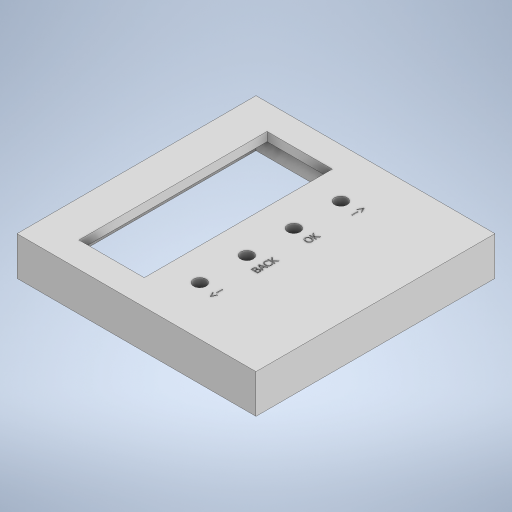
# Autodesk Inventor part: cover pcb
Saved by Autodesk Inventor 2023 (Build 270158030, 158C)
## iProperties
Created: 2023-02-26
Part Number: cover pcb
Material: Generic
Document SubType Name: Modeling
Designer: fatih
Density: 1 g/cm^3
Appearance: Default
Author: fatih
Autodesk Inventor part; units mm, degrees
ref_plane "YZ Plane" through (0, 0, 0) normal (1, 0, 0) x (0, 1, 0)
ref_plane "XZ Plane" through (0, 0, 0) normal (0, 1, 0) x (-1, 0, 0)
ref_plane "XY Plane" through (0, 0, 0) normal (0, 0, 1) x (1, 0, 0)
sketch "Sketch1" plane through (0, 0, 0) normal (0, 1, 0) x (-1, 0, 0)
  line L0 (0, 0) -> (100, 0)
  line L1 (100, 0) -> (100, -100)
  line L2 (100, -100) -> (0, -100)
  line L3 (0, -100) -> (0, 0)
  dimension "d0" = 100
  dimension "d1" = 100
  constraints: 8 end point, 2 parallel, 1 horizontal, 1 perpendicular
  measures "d0" distance of L2.end L0.start
  measures "d1" distance of L0.start L0.end
extrude "Extrusion1" add sketch "Sketch1" along normal blind 13.5
sketch "Sketch2" plane through (0, 13.5, 0) normal (0, 1, 0) x (1, 0, 0)
  line L0 (-100, 100) -> (-100, 0) projected
  line L1 (0, 0) -> (0, 100) projected
  line L2 (-87.5, 50) -> (-87.5, 92.5)
  line L3 (-87.5, 92.5) -> (-87.5, 7.5)
  line L4 (-87.5, 7.5) -> (-58, 7.5)
  line L5 (-58, 7.5) -> (-58, 92.5)
  line L6 (-58, 92.5) -> (-87.5, 92.5)
  dimension "d4" = 42.5
  dimension "d5" = 85
  dimension "d6" = 29.5
  constraints: 10 end point, 3 perpendicular, 1 point on line, 1 vertical
  measures "d4" distance of L2.start L2.end
  measures "d5" distance of L2.end L3.end
  measures "d6" distance of L3.end L4.end
shell "Shell1" thickness 4 outward yes removed faces 1 at (-33.3333, 0, -33.3333)
extrude "Extrusion2" cut sketch "Sketch2" along normal blind 13.5
sketch "Sketch3" plane through (0, 17.5, 0) normal (0, 1, 0) x (1, 0, 0)
  line L0 (-58, 7.5) -> (-58, 92.5) projected
  line L1 (-58, 50) -> (0, 50)
  line L2 (0, 0) -> (0, 100) projected
  line L3 (-29, 50) -> (-58, 50)
  line L4 (-87.5, 7.5) -> (-58, 7.5) projected
  circle A0 centre (-43.5, 81.875) radius 2.85
  circle A1 centre (-43.5, 60.625) radius 2.85
  circle A2 centre (-43.5, 18.125) radius 2.85
  circle A3 centre (-43.5, 39.375) radius 2.85
  dimension "d10" = 5.7
  dimension "d11" = 5.7
  constraints: 4 centre point, 4 end point, 3 midpoint, 2 symmetric about line, 1 collinear, 2 other
  measures "d10" diameter of A0
  measures "d11" diameter of A1
extrude "Extrusion3" cut sketch "Sketch3" against normal blind 13.5
sketch "Sketch5" plane through (0, 17.5, 0) normal (0, 1, 0) x (1, 0, 0)
  circle A0 centre (-43.5, 18.125) radius 2.85 projected
  line L0 (-40.65, 18.125) -> (-40.65, 81.875)
  circle A1 centre (-43.5, 81.875) radius 2.85 projected
  line L1 (-30.65, 18.125) -> (-30.65, 81.875)
  line L2 (-40.65, 81.875) -> (-40.65, 18.125)
  line L3 (-30.65, 15.275) -> (-30.65, 84.725)
  line L4 (-40.65, 84.725) -> (-40.65, 15.275)
  line L5 (-36.861, 14.6566) -> (-36.861, 20.7501) construction
  line L6 (-36.861, 20.7501) -> (-34.517, 20.7501) construction
  line L7 (-34.517, 20.7501) -> (-34.517, 14.6566) construction
  line L8 (-34.517, 14.6566) -> (-36.861, 14.6566) construction
  line L9 (-36.7452, 78.7325) -> (-36.7452, 84.8261) construction
  line L10 (-36.7452, 84.8261) -> (-34.4012, 84.8261) construction
  line L11 (-34.4012, 84.8261) -> (-34.4012, 78.7325) construction
  line L12 (-34.4012, 78.7325) -> (-36.7452, 78.7325) construction
  line L13 (-37.2991, 57.9723) -> (-37.2991, 63.4039) construction
  line L14 (-37.2991, 63.4039) -> (-34.1227, 63.4039) construction
  line L15 (-34.1227, 63.4039) -> (-34.1227, 57.9723) construction
  line L16 (-34.1227, 57.9723) -> (-37.2991, 57.9723) construction
  line L17 (-37.2212, 34.5686) -> (-37.2212, 44.5351) construction
  line L18 (-37.2212, 44.5351) -> (-33.6501, 44.5351) construction
  line L19 (-33.6501, 44.5351) -> (-33.6501, 34.5686) construction
  line L20 (-33.6501, 34.5686) -> (-37.2212, 34.5686) construction
  line L21 (-40.65, 84.725) -> (-40.65, 12.725)
  line L22 (-30.65, 12.725) -> (-30.65, 84.725)
  line L23 (-30.65, 12.725) -> (-30.65, 86.725)
  line L24 (-30.65, 86.725) -> (-40.65, 86.725)
  line L25 (-40.65, 86.725) -> (-40.65, 12.725)
  circle A2 centre (-43.5, 39.375) radius 2.85 projected
  circle A3 centre (-43.5, 60.625) radius 2.85 projected
  line L26 (-34.517, 17.2674) -> (-35.5668, 15.0691)
  line L27 (-35.5668, 15.0691) -> (-35.8113, 15.0691)
  line L28 (-35.8113, 15.0691) -> (-36.861, 17.2674)
  line L29 (-36.861, 17.2674) -> (-36.498, 17.2674)
  line L30 (-36.498, 17.2674) -> (-35.6903, 15.5631)
  line L31 (-35.6903, 15.5631) -> (-34.8801, 17.2674)
  line L32 (-34.8801, 17.2674) -> (-34.517, 17.2674)
  line L33 (-35.505, 19.0458) -> (-35.505, 17.8923)
  line L34 (-35.505, 17.8923) -> (-35.8755, 17.8923)
  line L35 (-35.8755, 17.8923) -> (-35.8755, 19.0458)
  line L36 (-35.8755, 19.0458) -> (-35.505, 19.0458)
  line L37 (-35.505, 20.5673) -> (-35.505, 19.4138)
  line L38 (-35.505, 19.4138) -> (-35.8755, 19.4138)
  line L39 (-35.8755, 19.4138) -> (-35.8755, 20.5673)
  line L40 (-35.8755, 20.5673) -> (-35.505, 20.5673)
  spline S0 degree 2 poles (-35.055, 36.9448) (-34.8278, 36.9448) (-34.4795, 36.7719) (-34.3659, 36.6286) knots 0 0 0 1 2 2 2
  spline S1 degree 2 poles (-34.3659, 36.6286) (-34.2325, 36.4557) (-34.1189, 36.063) (-34.1189, 35.7518) knots 0 0 0 1 2 2 2
  line L41 (-34.1189, 35.7518) -> (-34.1189, 34.8774)
  line L42 (-34.1189, 34.8774) -> (-37.1669, 34.8774)
  line L43 (-37.1669, 34.8774) -> (-37.1669, 35.6851)
  spline S2 degree 2 poles (-37.1669, 35.6851) (-37.1669, 36.0111) (-37.1249, 36.3371) (-37.0434, 36.4853) knots 0 0 0 1 2 2 2
  spline S3 degree 2 poles (-37.0434, 36.4853) (-36.9569, 36.6508) (-36.6729, 36.8015) (-36.4802, 36.8015) knots 0 0 0 1 2 2 2
  spline S4 degree 2 poles (-36.4802, 36.8015) (-36.2653, 36.8015) (-35.9245, 36.5743) (-35.8281, 36.3742) knots 0 0 0 1 2 2 2
  line L44 (-35.8281, 36.3742) -> (-35.8133, 36.3742)
  spline S5 degree 2 poles (-35.8133, 36.3742) (-35.7392, 36.6459) (-35.3465, 36.9448) (-35.055, 36.9448) knots 0 0 0 1 2 2 2
  spline S6 degree 2 poles (-35.0377, 36.5224) (-35.2106, 36.5224) (-35.4329, 36.4236) (-35.512, 36.2754) knots 0 0 0 1 2 2 2
  spline S7 degree 2 poles (-35.512, 36.2754) (-35.5614, 36.1791) (-35.591, 35.9518) (-35.591, 35.7419) knots 0 0 0 1 2 2 2
  line L45 (-35.591, 35.7419) -> (-35.591, 35.2825)
  line L46 (-35.591, 35.2825) -> (-34.4647, 35.2825)
  line L47 (-34.4647, 35.2825) -> (-34.4647, 35.611)
  spline S8 degree 2 poles (-34.4647, 35.611) (-34.4647, 35.8777) (-34.5141, 36.184) (-34.5931, 36.3026) knots 0 0 0 1 2 2 2
  spline S9 degree 2 poles (-34.5931, 36.3026) (-34.6746, 36.4162) (-34.8772, 36.5224) (-35.0377, 36.5224) knots 0 0 0 1 2 2 2
  spline S10 degree 2 poles (-36.4234, 36.3791) (-36.5321, 36.3791) (-36.6951, 36.305) (-36.742, 36.2235) knots 0 0 0 1 2 2 2
  spline S11 degree 2 poles (-36.742, 36.2235) (-36.7964, 36.1247) (-36.8211, 35.8851) (-36.8211, 35.6702) knots 0 0 0 1 2 2 2
  line L48 (-36.8211, 35.6702) -> (-36.8211, 35.2825)
  line L49 (-36.8211, 35.2825) -> (-35.9294, 35.2825)
  line L50 (-35.9294, 35.2825) -> (-35.9294, 35.7419)
  spline S12 degree 2 poles (-35.9294, 35.7419) (-35.9294, 35.9321) (-35.9689, 36.1124) (-36.0307, 36.2087) knots 0 0 0 1 2 2 2
  spline S13 degree 2 poles (-36.0307, 36.2087) (-36.09, 36.3026) (-36.2801, 36.3791) (-36.4234, 36.3791) knots 0 0 0 1 2 2 2
  line L51 (-34.1189, 37.0189) -> (-37.1669, 38.0464)
  line L52 (-37.1669, 38.0464) -> (-37.1669, 38.5453)
  line L53 (-37.1669, 38.5453) -> (-34.1189, 39.5729)
  line L54 (-34.1189, 39.5729) -> (-34.1189, 39.1456)
  line L55 (-34.1189, 39.1456) -> (-34.971, 38.8689)
  line L56 (-34.971, 38.8689) -> (-34.971, 37.7055)
  line L57 (-34.971, 37.7055) -> (-34.1189, 37.4289)
  line L58 (-34.1189, 37.4289) -> (-34.1189, 37.0189)
  line L59 (-35.3168, 38.7578) -> (-36.7519, 38.286)
  line L60 (-36.7519, 38.286) -> (-35.3168, 37.8167)
  line L61 (-35.3168, 37.8167) -> (-35.3168, 38.7578)
  spline S14 degree 2 poles (-34.0645, 41.0524) (-34.0645, 40.756) (-34.2646, 40.2546) (-34.4647, 40.0718) knots 0 0 0 1 2 2 2
  spline S15 degree 2 poles (-34.4647, 40.0718) (-34.6623, 39.889) (-35.2551, 39.689) (-35.6404, 39.689) knots 0 0 0 1 2 2 2
  spline S16 degree 2 poles (-35.6404, 39.689) (-36.0233, 39.689) (-36.5914, 39.8841) (-36.8013, 40.0693) knots 0 0 0 1 2 2 2
  spline S17 degree 2 poles (-36.8013, 40.0693) (-37.0063, 40.2521) (-37.2212, 40.7511) (-37.2212, 41.0598) knots 0 0 0 1 2 2 2
  spline S18 degree 2 poles (-37.2212, 41.0598) (-37.2212, 41.213) (-37.1768, 41.4822) (-37.1422, 41.5958) knots 0 0 0 1 2 2 2
  spline S19 degree 2 poles (-37.1422, 41.5958) (-37.1101, 41.6946) (-37.0187, 41.8996) (-36.9643, 42.0009) knots 0 0 0 1 2 2 2
  line L62 (-36.9643, 42.0009) -> (-36.4753, 42.0009)
  line L63 (-36.4753, 42.0009) -> (-36.4753, 41.9688)
  spline S20 degree 2 poles (-36.4753, 41.9688) (-36.5247, 41.9144) (-36.663, 41.7465) (-36.7297, 41.6255) knots 0 0 0 1 2 2 2
  spline S21 degree 2 poles (-36.7297, 41.6255) (-36.7939, 41.5094) (-36.8754, 41.2352) (-36.8754, 41.0573) knots 0 0 0 1 2 2 2
  spline S22 degree 2 poles (-36.8754, 41.0573) (-36.8754, 40.8622) (-36.7149, 40.5139) (-36.5617, 40.383) knots 0 0 0 1 2 2 2
  spline S23 degree 2 poles (-36.5617, 40.383) (-36.4061, 40.2546) (-35.9343, 40.1113) (-35.6404, 40.1113) knots 0 0 0 1 2 2 2
  spline S24 degree 2 poles (-35.6404, 40.1113) (-35.3267, 40.1113) (-34.8747, 40.262) (-34.7191, 40.3929) knots 0 0 0 1 2 2 2
  spline S25 degree 2 poles (-34.7191, 40.3929) (-34.5684, 40.5214) (-34.4153, 40.8647) (-34.4153, 41.0573) knots 0 0 0 1 2 2 2
  spline S26 degree 2 poles (-34.4153, 41.0573) (-34.4153, 41.2327) (-34.5017, 41.5316) (-34.566, 41.6477) knots 0 0 0 1 2 2 2
  spline S27 degree 2 poles (-34.566, 41.6477) (-34.6302, 41.7588) (-34.7636, 41.9243) (-34.8105, 41.9713) knots 0 0 0 1 2 2 2
  line L64 (-34.8105, 41.9713) -> (-34.8105, 42.0009)
  line L65 (-34.8105, 42.0009) -> (-34.3264, 42.0009)
  spline S28 degree 2 poles (-34.3264, 42.0009) (-34.2794, 41.8996) (-34.193, 41.7218) (-34.1535, 41.5958) knots 0 0 0 1 2 2 2
  spline S29 degree 2 poles (-34.1535, 41.5958) (-34.109, 41.4624) (-34.0645, 41.2352) (-34.0645, 41.0524) knots 0 0 0 1 2 2 2
  line L66 (-34.1189, 44.6018) -> (-34.1189, 44.0757)
  line L67 (-34.1189, 44.0757) -> (-35.5367, 42.9617)
  line L68 (-35.5367, 42.9617) -> (-35.3366, 42.7839)
  line L69 (-35.3366, 42.7839) -> (-34.1189, 42.7839)
  line L70 (-34.1189, 42.7839) -> (-34.1189, 42.3788)
  line L71 (-34.1189, 42.3788) -> (-37.1669, 42.3788)
  line L72 (-37.1669, 42.3788) -> (-37.1669, 42.7839)
  line L73 (-37.1669, 42.7839) -> (-35.7664, 42.7839)
  line L74 (-35.7664, 42.7839) -> (-37.1669, 44.0337)
  line L75 (-37.1669, 44.0337) -> (-37.1669, 44.5277)
  line L76 (-37.1669, 44.5277) -> (-35.8059, 43.2655)
  line L77 (-35.8059, 43.2655) -> (-34.1189, 44.6018)
  spline S30 degree 2 poles (-36.8866, 60.4374) (-36.6841, 60.6103) (-36.0913, 60.8029) (-35.7109, 60.8029) knots 0 0 0 1 2 2 2
  spline S31 degree 2 poles (-35.7109, 60.8029) (-35.3404, 60.8029) (-34.7402, 60.6152) (-34.5377, 60.4374) knots 0 0 0 1 2 2 2
  spline S32 degree 2 poles (-34.5377, 60.4374) (-34.3252, 60.2497) (-34.1227, 59.7532) (-34.1227, 59.4543) knots 0 0 0 1 2 2 2
  spline S33 degree 2 poles (-34.1227, 59.4543) (-34.1227, 59.1456) (-34.3326, 58.6516) (-34.5377, 58.4712) knots 0 0 0 1 2 2 2
  spline S34 degree 2 poles (-34.5377, 58.4712) (-34.7402, 58.2959) (-35.3355, 58.1081) (-35.7109, 58.1081) knots 0 0 0 1 2 2 2
  spline S35 degree 2 poles (-35.7109, 58.1081) (-36.0938, 58.1081) (-36.6767, 58.2983) (-36.8866, 58.4737) knots 0 0 0 1 2 2 2
  spline S36 degree 2 poles (-36.8866, 58.4737) (-37.0892, 58.6516) (-37.2991, 59.148) (-37.2991, 59.4543) knots 0 0 0 1 2 2 2
  spline S37 degree 2 poles (-37.2991, 59.4543) (-37.2991, 59.7655) (-37.0818, 60.2645) (-36.8866, 60.4374) knots 0 0 0 1 2 2 2
  spline S38 degree 2 poles (-35.7109, 60.3806) (-36.0123, 60.3806) (-36.4791, 60.2497) (-36.6322, 60.1311) knots 0 0 0 1 2 2 2
  spline S39 degree 2 poles (-36.6322, 60.1311) (-36.7903, 60.0101) (-36.9484, 59.6692) (-36.9484, 59.4568) knots 0 0 0 1 2 2 2
  spline S40 degree 2 poles (-36.9484, 59.4568) (-36.9484, 59.2369) (-36.7952, 58.906) (-36.6322, 58.78) knots 0 0 0 1 2 2 2
  spline S41 degree 2 poles (-36.6322, 58.78) (-36.4766, 58.659) (-36.0073, 58.5305) (-35.7109, 58.5305) knots 0 0 0 1 2 2 2
  spline S42 degree 2 poles (-35.7109, 58.5305) (-35.1107, 58.5305) (-34.4734, 59.0344) (-34.4734, 59.4568) knots 0 0 0 1 2 2 2
  spline S43 degree 2 poles (-34.4734, 59.4568) (-34.4734, 59.8791) (-35.1107, 60.3806) (-35.7109, 60.3806) knots 0 0 0 1 2 2 2
  line L78 (-34.1869, 63.4706) -> (-34.1869, 62.9444)
  line L79 (-34.1869, 62.9444) -> (-35.6047, 61.8305)
  line L80 (-35.6047, 61.8305) -> (-35.4046, 61.6526)
  line L81 (-35.4046, 61.6526) -> (-34.1869, 61.6526)
  line L82 (-34.1869, 61.6526) -> (-34.1869, 61.2475)
  line L83 (-34.1869, 61.2475) -> (-37.2349, 61.2475)
  line L84 (-37.2349, 61.2475) -> (-37.2349, 61.6526)
  line L85 (-37.2349, 61.6526) -> (-35.8344, 61.6526)
  line L86 (-35.8344, 61.6526) -> (-37.2349, 62.9024)
  line L87 (-37.2349, 62.9024) -> (-37.2349, 63.3965)
  line L88 (-37.2349, 63.3965) -> (-35.8739, 62.1343)
  line L89 (-35.8739, 62.1343) -> (-34.1869, 63.4706)
  line L90 (-35.3892, 80.0713) -> (-35.3892, 78.9178)
  line L91 (-35.3892, 78.9178) -> (-35.7597, 78.9178)
  line L92 (-35.7597, 78.9178) -> (-35.7597, 80.0713)
  line L93 (-35.7597, 80.0713) -> (-35.3892, 80.0713)
  line L94 (-35.3892, 81.5928) -> (-35.3892, 80.4393)
  line L95 (-35.3892, 80.4393) -> (-35.7597, 80.4393)
  line L96 (-35.7597, 80.4393) -> (-35.7597, 81.5928)
  line L97 (-35.7597, 81.5928) -> (-35.3892, 81.5928)
  line L98 (-35.451, 84.4136) -> (-34.4012, 82.2153)
  line L99 (-34.4012, 82.2153) -> (-34.7643, 82.2153)
  line L100 (-34.7643, 82.2153) -> (-35.5745, 83.9196)
  line L101 (-35.5745, 83.9196) -> (-36.3822, 82.2153)
  line L102 (-36.3822, 82.2153) -> (-36.7452, 82.2153)
  line L103 (-36.7452, 82.2153) -> (-35.6955, 84.4136)
  line L104 (-35.6955, 84.4136) -> (-35.451, 84.4136)
  point P0 (0, 0)
  dimension "d14" = 10
  dimension "d15" = 72
  dimension "d16" = 74
  constraints: 20 end point, 4 parallel, 2 horizontal alignment, 2 point on line, 1 vertical, 10 other
  measures "d14" distance of L2.start L1.end
  measures "d15" distance of L21.start L21.end
  measures "d16" distance of L23.start L23.end
emboss "Emboss1" sketch "Sketch5" operation cut depth 1 direction (0, -1, 0) contours L26 L27 L28 L29 L30 L31 L32 | L33 L34 L35 L36 | L37 L38 L39 L40 | S0 S1 L41 L42 L43 S2 S3 S4 L44 S5 | L51 L52 L53 L54 L55 L56 L57 L58 | S14 S15 S16 S17 S18 S19 L62 L63 S20 S21 S22 S23 S24 S25 S26 S27 L64 L65 S28 S29 | L66 L67 L68 L69 L70 L71 L72 L73 L74 L75 L76 L77 | S30 S31 S32 S33 S34 S35 S36 S37 | L78 L79 L80 L81 L82 L83 L84 L85 L86 L87 L88 L89 | L90 L91 L92 L93 | L94 L95 L96 L97 | L98 L99 L100 L101 L102 L103 L104
body "Solid1"
